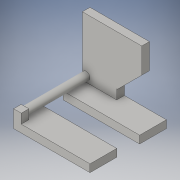
# Autodesk Inventor part: handbase
Saved by Autodesk Inventor 2016 (Build 200138000, 138)
## iProperties
Created: 2018-01-10
Part Number: handbase
Material: Generic
Document SubType Name: Modeling
Designer: New User
Density: 1 g/cm^3
Appearance: Default
Author: New User
Autodesk Inventor part; units mm, degrees
ref_plane "YZ Plane" through (0, 0, 0) normal (1, 0, 0) x (0, 1, 0)
ref_plane "XZ Plane" through (0, 0, 0) normal (0, 1, 0) x (-1, 0, 0)
ref_plane "XY Plane" through (0, 0, 0) normal (0, 0, 1) x (1, 0, 0)
sketch "Sketch1" plane through (0, 0, 0) normal (0, 1, 0) x (-1, 0, 0)
  line L0 (0, 0) -> (-254, 0)
  line L1 (-254, 0) -> (-254, 88.9)
  line L2 (-254, 88.9) -> (0, 88.9)
  line L3 (0, 88.9) -> (0, 0)
  line L4 (0, -76.2) -> (-254, -76.2)
  line L5 (-254, -76.2) -> (-254, -165.1)
  line L6 (-254, -165.1) -> (0, -165.1)
  line L7 (0, -165.1) -> (0, -76.2)
  dimension "d0" = 88.9
  dimension "d1" = 254
  dimension "d2" = 254
  dimension "d3" = 88.9
  dimension "d4" = 76.2
  constraints: 16 end point, 4 parallel, 2 horizontal, 2 perpendicular
  measures "d0" distance of L2.end L0.start
  measures "d1" distance of L1.end L2.end
  measures "d2" distance of L5.end L6.end
  measures "d3" distance of L6.end L4.start
  measures "d4" distance between parallel lines of L4 L0
extrude "Extrusion1" add sketch "Sketch1" along normal blind 25.4
sketch "Sketch2" plane through (0, 25.4, 0) normal (0, 1, 0) x (1, 0, 0)
  line L0 (0, -88.9) -> (25.4, -88.9)
  line L1 (25.4, -88.9) -> (25.4, -63.5)
  line L2 (25.4, -63.5) -> (0, -63.5)
  line L3 (0, -63.5) -> (0, -88.9)
  line L4 (0, 165.1) -> (114.3, 165.1)
  line L5 (114.3, 165.1) -> (114.3, 139.7)
  line L6 (114.3, 139.7) -> (0, 139.7)
  line L7 (0, 139.7) -> (0, 165.1)
  point P0 (25.4, 139.7)
  dimension "d7" = 25.4
  dimension "d17" = 114.3
  dimension "d18" = 25.4
  constraints: 16 end point, 4 parallel, 2 horizontal, 2 perpendicular, 1 point on line
  measures "d7" distance of L2.end L0.start
  measures "d17" distance of L4.start L4.end
  measures "d18" distance of L6.end L4.start
extrude "Extrusion2" add sketch "Sketch2" along normal blind 31.75
sketch "Sketch3" plane through (0, 0, 88.9) normal (0, 0, 1) x (1, 0, 0)
  circle A0 centre (12.7, 44.45) radius 12.7
  line L0 (25.4, 57.15) -> (0, 57.15) projected
  point P0 (0, 0)
  dimension "d13" = 12.7
  dimension "d14" = 25.4
  constraints: 1 centre point
  measures "d13" distance from line of L0 A0.centre
  measures "d14" diameter of A0
extrude "Extrusion3" add sketch "Sketch3" against normal blind 242.8875
sketch "Sketch4" plane through (0, 57.15, 0) normal (0, 1, 0) x (1, 0, 0)
  line L0 (0, 165.1) -> (0, 76.2) projected
  line L1 (0, 165.1) -> (197.3764, 165.1)
  line L2 (197.3764, 165.1) -> (197.3764, 139.7)
  line L3 (197.3764, 139.7) -> (0, 139.7)
  line L4 (0, 139.7) -> (0, 165.1)
  point P0 (0, 0)
  constraints: 8 end point, 2 parallel, 1 horizontal, 1 perpendicular
extrude "Extrusion4" add sketch "Sketch4" along normal blind 165.1
chamfer "Chamfer1" distance 80.9625 angle 45 1 edges at (197.3764, 57.15, -152.4)
body "Solid1"
